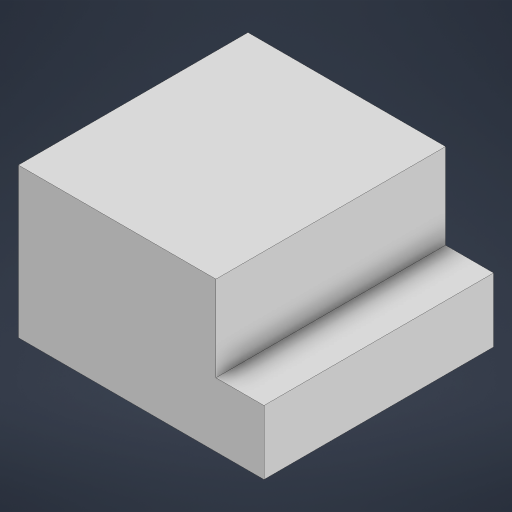
# Autodesk Inventor part: chasis
Saved by Autodesk Inventor 2023 (Build 270158000, 158)
## iProperties
Created: 2022-08-21
Part Number: chasis
Material: Generic
Document SubType Name: Modeling
Designer: marat
Density: 1 g/cm^3
Appearance: Default
Author: marat
Autodesk Inventor part; units mm, degrees
ref_plane "YZ Plane" through (0, 0, 0) normal (1, 0, 0) x (0, 1, 0)
ref_plane "XZ Plane" through (0, 0, 0) normal (0, 1, 0) x (-1, 0, 0)
ref_plane "XY Plane" through (0, 0, 0) normal (0, 0, 1) x (1, 0, 0)
sketch "Sketch1" plane through (0, 0, 0) normal (0, 1, 0) x (-1, 0, 0)
  line L0 (115, 107.5) -> (-115, 107.5)
  line L1 (-115, 107.5) -> (-115, -107.5)
  line L2 (-115, -107.5) -> (115, -107.5)
  line L3 (115, -107.5) -> (115, 107.5)
  line L4 (115, 107.5) -> (-115, -107.5) construction
  line L5 (-115, 107.5) -> (115, -107.5) construction
  point P0 (0, 0)
  dimension "d0" = 230
  dimension "d1" = 215
  constraints: 12 end point, 2 midpoint, 2 parallel, 1 horizontal, 1 perpendicular
  measures "d0" distance of L2.end L1.end
  measures "d1" distance of L1.end L0.end
extrude "Extrusion1" add sketch "Sketch1" along normal blind 60
sketch "Sketch2" plane through (0, 60, 0) normal (0, 1, 0) x (1, 0, 0)
  line L0 (-115, 107.5) -> (-115, -107.5) projected
  line L1 (115, 107.5) -> (-115, 107.5) projected
  line L2 (-115, -107.5) -> (70, -107.5)
  line L3 (70, -107.5) -> (70, 107.5)
  line L4 (70, 107.5) -> (-115, 107.5)
  line L5 (-115, 107.5) -> (-115, -107.5)
  point P0 (0, 0)
  dimension "d4" = 185
  constraints: 8 end point, 2 parallel, 1 horizontal, 1 perpendicular, 1 point on line
  measures "d4" distance of L4.end L3.end
extrude "Extrusion2" add sketch "Sketch2" along normal blind 80
body "Solid1"
